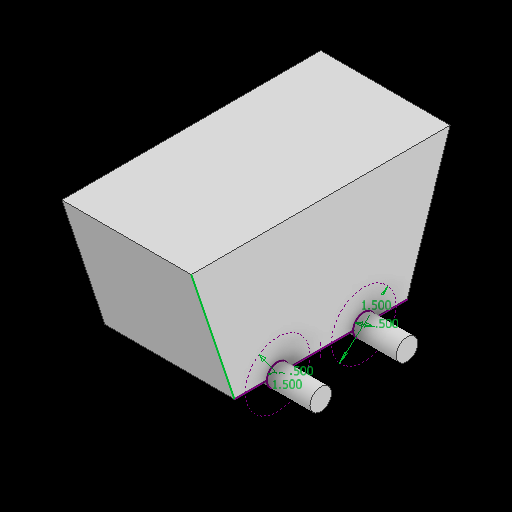
# Autodesk Inventor part: CartMK1
Saved by Autodesk Inventor 2025 (Build 290162000, 162)
## iProperties
Created: 2025-03-04
Part Number: CartMK1
Material: Generic
Document SubType Name: Modeling
Designer: Trevor
Density: 1 g/cm^3
Appearance: Default
Author: Trevor
Autodesk Inventor part; units mm, degrees
ref_plane "YZ Plane" through (0, 0, 0) normal (1, 0, 0) x (0, 1, 0)
ref_plane "XZ Plane" through (0, 0, 0) normal (0, 1, 0) x (-1, 0, 0)
ref_plane "XY Plane" through (0, 0, 0) normal (0, 0, 1) x (1, 0, 0)
sketch "Sketch1" plane through (0, 0, 0) normal (1, 0, 0) x (0, 1, 0)
  line L0 (0, 0) -> (0, -101.6)
  line L1 (0, -50.8) -> (76.2, -50.8) construction
  line L2 (76.2, -50.8) -> (76.2, 25.4)
  line L3 (76.2, 25.4) -> (0, 0)
  line L4 (76.2, -50.8) -> (76.2, -127)
  line L5 (76.2, -127) -> (0, -101.6)
  dimension "d0" = 101.6
  dimension "d1" = 76.2
  dimension "d2" = 76.2
  dimension "d3" = 76.2
  constraints: 12 end point, 1 horizontal, 1 midpoint, 1 perpendicular, 1 point on line, 1 vertical
  measures "d0" distance of L0.start L0.end
  measures "d1" distance of L1.start L1.end
  measures "d2" distance of L1.end L2.end
  measures "d3" distance of L1.end L4.end
extrude "Extrusion1" add sketch "Sketch1" along normal mid plane 76.2
sketch "Sketch3" plane through (38.1, 0, 0) normal (1, 0, 0) x (0, 0, -1)
  line L0 (0, 0) -> (101.6, 0) projected
  line L1 (-25.4, 76.2) -> (0, 0) projected
  line L2 (0, 0) -> (50.8, 0)
  line L3 (50.8, 0) -> (101.6, 0)
  circle A0 centre (25.4, 0) radius 19.05 construction
  circle A1 centre (76.2, 0) radius 19.05 construction
  circle A2 centre (25.4, 0) radius 6.35
  circle A3 centre (76.2, 0) radius 6.35
  point P0 (31.75, 0)
  point P1 (19.05, 0)
  point P2 (82.55, 0)
  point P3 (69.85, 0)
  dimension "d7" = 38.1
  dimension "d8" = 38.1
  dimension "d9" = 12.7
  dimension "d10" = 12.7
  constraints: 4 centre point, 4 coincident, 4 end point, 3 midpoint, 1 collinear, 1 horizontal
  measures "d7" diameter of A0
  measures "d8" diameter of A1
  measures "d9" diameter of A2
  measures "d10" diameter of A3
extrude "Extrusion2" add sketch "Sketch3" against normal up to surface (76.2 mm away) contours L0 A2 | L0 A3 picked at (25.6551, -2.1012) picked at (75.9449, -2.1012)
extrude "Extrusion3" add sketch "Sketch3" along normal blind 25.4
sketch "Sketch4" plane through (-38.1, 0, 0) normal (-1, 0, 0) x (0, 0, 1)
  line L0 (0, 0) -> (25.4, 76.2) projected
  line L1 (25.4, 76.2) -> (-127, 76.2) projected
  line L2 (-127, 76.2) -> (-101.6, 0) projected
  line L3 (-101.6, 0) -> (-82.55, 0) projected
  arc A0 (-82.55, 0) -> (-69.85, 0) centre (-76.2, 0) ccw projected
  line L4 (-69.85, 0) -> (-31.75, 0) projected
  arc A1 (-31.75, 0) -> (-19.05, 0) centre (-25.4, 0) ccw projected
  line L5 (-19.05, 0) -> (0, 0) projected
  line L6 (0, 0) -> (25.4, 76.2) projected
  line L7 (25.4, 76.2) -> (-127, 76.2) projected
  line L8 (-127, 76.2) -> (-101.6, 0) projected
  line L9 (-101.6, 0) -> (-82.55, 0) projected
  arc A2 (-82.55, 0) -> (-69.85, 0) centre (-76.2, 0) ccw projected
  line L10 (-69.85, 0) -> (-31.75, 0) projected
  arc A3 (-31.75, 0) -> (-19.05, 0) centre (-25.4, 0) ccw projected
  line L11 (-19.05, 0) -> (0, 0) projected
  circle A4 centre (-76.2, 0) radius 6.35
  circle A5 centre (-25.4, 0) radius 6.35
  point P0 (-69.85, 0)
  point P1 (-19.05, 0)
  constraints: 2 coincident, 6 other
extrude "Extrusion4" add sketch "Sketch4" along normal blind 25.4 contours A1 A5 | A0 A4
body "Solid1"
